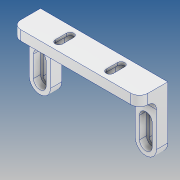
# Autodesk Inventor part: 103.007.01_Einstellwinkel
Saved by Autodesk Inventor 2021 (Build 250183000, 183)
## iProperties
Created: 2021-11-03
Part Number: 103.007.01_Einstellwinkel
Material: Aluminium 6061
Document SubType Name: Modeling
Designer: Sebastian Seewald
Density: 2.7 g/cm^3
Appearance: Aluminium - flach
Mass: 47.3995 g
Surface Area: 90.6032 cm^2
Volume: 17.5554 cm^3
Author: Sebastian Seewald
Title: Haltekonsole
Autodesk Inventor part; units mm, degrees
ref_plane "YZ Plane" through (0, 0, 0) normal (1, 0, 0) x (0, 1, 0)
ref_plane "XZ Plane" through (0, 0, 0) normal (0, 1, 0) x (-1, 0, 0)
ref_plane "XY Plane" through (0, 0, 0) normal (0, 0, 1) x (1, 0, 0)
sketch "Skizze1" plane through (0, 0, 0) normal (0, 0, 1) x (1, 0, 0)
  line L0 (-45, 2.5) -> (45, 2.5)
  line L1 (45, 2.5) -> (45, -4.5)
  line L2 (45, -4.5) -> (-45, -4.5)
  line L3 (-45, -4.5) -> (-45, 2.5)
  point P0 (0, 0)
  dimension "d0" = 7
  dimension "d1" = 90
  dimension "d2" = 45
  dimension "d3" = 2.5
  constraints: 8 end point, 2 parallel, 1 horizontal, 1 perpendicular
  measures "d0" distance between parallel lines of L2 L0
  measures "d1" distance between parallel lines of L1 L3
  measures "d2" distance from line of point (0, 0) L3
  measures "d3" distance from line of point (0, 0) L0
extrude "Extrusion1" add sketch "Skizze1" along normal blind 20
sketch "Skizze2" plane through (0, 0, 0) normal (0, 0, -1) x (-1, 0, 0)
  line L0 (-45, 2.5) -> (45, 2.5) projected
  line L1 (37.5, -42.5) -> (37.5, -42.5)
  line L2 (30, -35) -> (30, 2.5)
  line L3 (30, 2.5) -> (45, 2.5)
  line L4 (45, 2.5) -> (45, -35)
  line L5 (45, 2.5) -> (45, -4.5) projected
  arc A0 (30, -35) -> (37.5, -42.5) centre (37.5, -35) ccw
  arc A1 (37.5, -42.5) -> (45, -35) centre (37.5, -35) ccw
  line L6 (37.5, -35) -> (37.5, -20) construction
  line L7 (40.1, -35) -> (40.1, -20)
  line L8 (34.9, -20) -> (34.9, -35)
  arc A2 (34.9, -35) -> (40.1, -35) centre (37.5, -35) ccw
  arc A3 (40.1, -20) -> (34.9, -20) centre (37.5, -20) ccw
  point P0 (0, 0)
  point P1 (37.5, -27.5)
  dimension "d8" = 45
  dimension "d9" = 7.5
  dimension "d14" = 5.2
  dimension "d15" = 15
  dimension "d16" = 4.9
  dimension "d38" = 4.9
  constraints: 16 end point, 8 point on circle, 8 tangent, 4 centre point, 3 parallel, 1 coincident, 1 collinear, 1 concentric, 1 horizontal, 1 midpoint, 1 perpendicular, 1 point on line, 1 vertical
  measures "d8" distance between parallel lines of L0 L1
  measures "d9" radius of A0
  measures "d14" distance between parallel lines of L8 L7
  measures "d15" distance of L6.start L6.end
  measures "d16" distance between parallel lines of L4 L7
  measures "d38" distance between parallel lines of L8 L2
extrude "Extrusion2" add sketch "Skizze2" against normal blind 8
fillet "Rundung2" radius 6 2 edges at (-30, -4.5, 4) (-37.5, -4.5, 8)
sketch "Skizze3" plane through (0, 0, 8) normal (0, 0, 1) x (1, 0, 0)
  line L0 (-34.9, -20) -> (-34.9, -35) projected
  arc A0 (-34.9, -20) -> (-40.1, -20) centre (-37.5, -20) ccw projected
  line L1 (-40.1, -35) -> (-40.1, -20) projected
  arc A1 (-40.1, -35) -> (-34.9, -35) centre (-37.5, -35) ccw projected
  arc A2 (-33, -20) -> (-42, -20) centre (-37.5, -20) ccw
  line L2 (-33, -20) -> (-33, -35)
  arc A3 (-42, -35) -> (-33, -35) centre (-37.5, -35) ccw
  line L3 (-42, -35) -> (-42, -20)
  point P0 (0, 0)
  dimension "d20" = 9
  constraints: 4 end point, 4 point on circle, 2 centre point, 3 other
  measures "d20" distance between parallel lines of L3 L2
extrude "Extrusion3" cut sketch "Skizze3" along normal blind 5 and the other way blind 5
mirror "Spiegeln1" about plane through (0, 0, 0) normal (1, 0, 0) of "Extrusion2", "Rundung2", "Extrusion3"
sketch "Skizze4" plane through (-24, -4.5, 0) normal (0, -1, 0) x (1, 0, 0)
  line L0 (6, 14) -> (6, 6) construction
  line L1 (3.4, 14) -> (3.4, 6)
  line L2 (8.6, 6) -> (8.6, 14)
  arc A0 (8.6, 14) -> (3.4, 14) centre (6, 14) ccw
  arc A1 (3.4, 6) -> (8.6, 6) centre (6, 6) ccw
  line L3 (0, 0) -> (48, 0) projected
  line L4 (-21, 20) -> (69, 20) projected
  point P0 (24, 0)
  point P1 (6, 10)
  point P2 (52, 0)
  point P3 (69, 0)
  point P4 (-15, 20)
  dimension "d26" = 5.2
  dimension "d27" = 8
  dimension "d29" = 6
  dimension "d30" = 18
  dimension "d39" = 6
  constraints: 8 end point, 4 point on circle, 4 tangent, 2 centre point, 1 midpoint, 1 parallel, 1 vertical
  measures "d26" distance between parallel lines of L1 L2
  measures "d27" distance of L0.start L0.end
  measures "d29" distance from line of L3 L0.end
  measures "d30" distance from line of L0 point (24, 0)
  measures "d39" distance from line of L4 L0.start
extrude "Extrusion4" cut sketch "Skizze4" against normal up to surface (7 mm away)
sketch "Skizze5" plane through (-24, -4.5, 0) normal (0, -1, 0) x (1, 0, 0)
  arc A0 (8.6, 14) -> (3.4, 14) centre (6, 14) ccw projected
  line L0 (3.4, 6) -> (3.4, 14) projected
  line L1 (8.6, 14) -> (8.6, 6) projected
  arc A1 (3.4, 6) -> (8.6, 6) centre (6, 6) ccw projected
  arc A2 (10.3, 14) -> (1.7, 14) centre (6, 14) ccw
  line L2 (10.3, 14) -> (10.3, 6)
  arc A3 (1.7, 6) -> (10.3, 6) centre (6, 6) ccw
  line L3 (1.7, 6) -> (1.7, 14)
  point P0 (24, 0)
  dimension "d33" = 8.6
  constraints: 4 end point, 4 point on circle, 2 centre point, 3 other
  measures "d33" distance between parallel lines of L3 L2
extrude "Extrusion5" cut sketch "Skizze5" against normal blind 5
mirror "Spiegeln2" about plane through (0, 0, 0) normal (1, 0, 0) of "Extrusion4", "Extrusion5"
fillet "Rundung7" radius 6 2 edges at (-45, -1, 20) (45, -1, 20)
